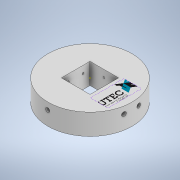
# Autodesk Inventor part: Base_V2a
Saved by Autodesk Inventor 2022 (Build 260153000, 153)
## iProperties
Created: 2022-06-15
Part Number: Base_V2a
Material: Generic
Document SubType Name: Modeling
Designer: Asus
Density: 1 g/cm^3
Appearance: Default
Author: Asus
Autodesk Inventor part; units mm, degrees
ref_plane "XZ Plane" through (0, 0, 0) normal (0, 1, 0) x (-1, 0, 0)
sketch "Sketch1" plane through (0, 0, 0) normal (0, 1, 0) x (-1, 0, 0)
  circle A0 centre (0, 0) radius 90
  dimension "d0" = 180
  constraints: 1 centre point, 1 coincident
  measures "d0" diameter of A0
extrude "Extrusion1" add sketch "Sketch1" along normal blind 25
sketch "Sketch2" plane through (0, 25, 0) normal (0, 1, 0) x (1, 0, 0)
  line L0 (-30.75, 30.75) -> (30.75, 30.75)
  line L1 (30.75, 30.75) -> (30.75, -30.75)
  line L2 (30.75, -30.75) -> (-30.75, -30.75)
  line L3 (-30.75, -30.75) -> (-30.75, 30.75)
  point P0 (0, 0)
  dimension "d3" = 61.5
  dimension "d4" = 61.5
  dimension "d5" = 30.75
  dimension "d6" = 30.75
  constraints: 8 end point, 2 parallel, 1 horizontal, 1 perpendicular
  measures "d3" distance of L0.end L1.end
  measures "d4" distance of L0.start L0.end
  measures "d5" distance from line of point (0, 0) L1
  measures "d6" distance from line of L0 point (0, 0)
extrude "Extrusion2" cut sketch "Sketch2" against normal blind 25
sketch "Sketch3" plane through (-30.75, 25, 30.75) normal (1, 0, 0) x (0, 0, -1)
  circle A0 centre (46.5, -15) radius 1.95
  circle A1 centre (15, -15) radius 1.95
  line L0 (61.5, -25) -> (0, -25) projected
  line L1 (61.5, 0) -> (61.5, -25) projected
  line L2 (0, 0) -> (0, -25) projected
  point P0 (30.75, -25)
  dimension "d9" = 3.9
  dimension "d10" = 3.9
  dimension "d11" = 10
  dimension "d12" = 10
  dimension "d13" = 15
  dimension "d14" = 15
  constraints: 2 centre point
  measures "d9" diameter of A1
  measures "d10" diameter of A0
  measures "d11" vertical distance of point (30.75, -25) A0.centre
  measures "d12" distance from line of L0 A1.centre
  measures "d13" distance from line of L1 A0.centre
  measures "d14" distance from line of L2 A1.centre
extrude "Extrusion3" cut sketch "Sketch3" along normal mid plane 300
sketch "Sketch4" plane through (-30.75, 25, -30.75) normal (0, 0, 1) x (1, 0, 0)
  circle A0 centre (30, -15) radius 1.95
  line L0 (61.5, -25) -> (0, -25) projected
  line L1 (0, 0) -> (0, -25) projected
  point P0 (30.75, -25)
  dimension "d17" = 10
  dimension "d18" = 30
  dimension "d19" = 3.9
  constraints: 1 centre point
  measures "d17" distance from line of L0 A0.centre
  measures "d18" distance from line of L1 A0.centre
  measures "d19" diameter of A0
extrude "Extrusion4" cut sketch "Sketch4" along normal mid plane 300
ref_plane "Work Plane1" through (90, 0, 0) normal (1, 0, 0) x (0, 1, 0)
sketch "Sketch5" plane through (90, 0, 0) normal (1, 0, 0) x (0, 1, 0)
  circle A0 centre (10, -15.75) radius 1.95 projected
  circle A1 centre (10, -15.75) radius 4.5
  circle A2 centre (10, 15.75) radius 1.95 projected
  circle A3 centre (10, 15.75) radius 4.5
  point P0 (0, 0)
  dimension "d23" = 9
  dimension "d24" = 9
  constraints: 2 centre point, 2 coincident
  measures "d23" diameter of A3
  measures "d24" diameter of A1
extrude "Extrusion5" cut sketch "Sketch5" against normal blind 40 contours A0 | A1 | A2 | A3
mirror "Mirror1" about plane through (0, 0, 0) normal (1, 0, 0) of "Extrusion5"
ref_plane "Work Plane2" through (0, 0, 90) normal (0, 0, 1) x (1, 0, 0)
sketch "Sketch6" plane through (0, 0, 90) normal (0, 0, 1) x (1, 0, 0)
  circle A0 centre (-0.75, 10) radius 1.95 projected
  circle A1 centre (-0.75, 10) radius 4.5
  point P0 (0, 0)
  dimension "d28" = 9
  constraints: 1 centre point, 1 coincident
  measures "d28" diameter of A1
extrude "Extrusion6" cut sketch "Sketch6" against normal blind 40 contours A0 | A1
mirror "Mirror2" about plane through (0, 0, 0) normal (0, 0, 1) of "Extrusion6"
sketch "Sketch7" plane through (0, 0, 0) normal (0, -1, 0) x (1, 0, 0)
  circle A0 centre (0, 0) radius 90
  line L0 (-30.75, 30.75) -> (30.75, 30.75) projected
  line L1 (-30.75, 30.75) -> (30.75, 30.75)
  line L2 (30.75, 30.75) -> (30.75, -30.75)
  line L3 (30.75, -30.75) -> (-30.75, -30.75)
  line L4 (-30.75, -30.75) -> (-30.75, 30.75)
  constraints: 8 end point, 2 parallel, 1 centre point, 1 coincident, 1 horizontal, 1 perpendicular
extrude "Extrusion7" add sketch "Sketch7" along normal blind 20
sketch "Sketch8" plane through (0, 25, 0) normal (0, 1, 0) x (1, 0, 0)
  line L0 (37.3786, -36.9077) -> (37.3786, 35.2103) construction
  line L1 (37.3786, 35.2103) -> (75.2405, 35.2103) construction
  line L2 (75.2405, 35.2103) -> (75.2405, -36.9077) construction
  line L3 (75.2405, -36.9077) -> (37.3786, -36.9077) construction
  point P0 (0, 0)
  constraints: 2 other
body "Solid1"
